Autodesk Fusion 360 part; units mm, degrees
(part 2 of 3)
sketch "Sketch5" plane through (0, 0, 0) normal (0, 0, -1) x (1, 0, 0)
  arc A0 (13.748372, 9.324199) -> (13.417296, 7.858359) centre (14.366478, 8.414284) ccw
  line L0 (13.748372, 9.324199) -> (13.998575, 9.494162)
  spline S0 degree 5 poles (13.998575, 9.494162) (14.006089, 9.499267) (14.020968, 9.509672) (14.042834, 9.52587) (14.071131, 9.54859) (14.10533, 9.578527) (14.138686, 9.609581) (14.171524, 9.641334) (14.204082, 9.673474) (14.236451, 9.70588) (14.26862, 9.738556) (14.300516, 9.771583) (14.33205, 9.805066) (14.363159, 9.839079) (14.39384, 9.873623) (14.424122, 9.908656) (14.454056, 9.944111) (14.483697, 9.97992) (14.513083, 10.016032) (14.542226, 10.052428) (14.571122, 10.089111) (14.599759, 10.126094) (14.628121, 10.163392) (14.656202, 10.201013) (14.684003, 10.238952) (14.711532, 10.277197) (14.7388, 10.315731) (14.76582, 10.35454) (14.792599, 10.39361) (14.819141, 10.432935) (14.845446, 10.472514) (14.871513, 10.512344) (14.897342, 10.552427) (14.922931, 10.59276) (14.948283, 10.63334) (14.9734, 10.674162) (14.998286, 10.71522) (15.022944, 10.756508) (15.047376, 10.798023) (15.071584, 10.83976) (15.095569, 10.881717) (15.119331, 10.923891) (15.142871, 10.966281) (15.16619, 11.008883) (15.189289, 11.051696) (15.212169, 11.094715) (15.234832, 11.137939) (15.257278, 11.181365) (15.279509, 11.224989) (15.301525, 11.268809) (15.323328, 11.312823) (15.344917, 11.357029) (15.366295, 11.401425) (15.38746, 11.446008) (15.408415, 11.490777) (15.429159, 11.53573) (15.449693, 11.580863) (15.470018, 11.626176) (15.490134, 11.671666) (15.510043, 11.717332) (15.529744, 11.763171) (15.549238, 11.809183) (15.568525, 11.855365) (15.587606, 11.901715) (15.606482, 11.948232) (15.625151, 11.994914) (15.643616, 12.041758) (15.661877, 12.088763) (15.679933, 12.135927) (15.697785, 12.18325) (15.715433, 12.230731) (15.72939, 12.268841) (15.739766, 12.297494) (15.746643, 12.316628) (15.750071, 12.326202) knots 0 0 0 0 0 0 0.01428571 0.02857143 0.04285714 0.05714286 0.07142857 0.08571429 0.1 0.11428571 0.12857143 0.14285714 0.15714286 0.17142857 0.18571429 0.2 0.21428571 0.22857143 0.24285714 0.25714286 0.27142857 0.28571429 0.3 0.31428571 0.32857143 0.34285714 0.35714286 0.37142857 0.38571429 0.4 0.41428571 0.42857143 0.44285714 0.45714286 0.47142857 0.48571429 0.5 0.51428571 0.52857143 0.54285714 0.55714286 0.57142857 0.58571429 0.6 0.61428571 0.62857143 0.64285714 0.65714286 0.67142857 0.68571429 0.7 0.71428571 0.72857143 0.74285714 0.75714286 0.77142857 0.78571429 0.8 0.81428571 0.82857143 0.84285714 0.85714286 0.87142857 0.88571429 0.9 0.91428571 0.92857143 0.94285714 0.95714286 0.97142857 0.98571429 1 1 1 1 1 1
  arc A1 (15.750071, 12.326202) -> (14.873911, 13.37037) centre (0, 0) ccw
  spline S1 degree 5 poles (11.780751, 12.137261) (11.787083, 12.143775) (11.799915, 12.15662) (11.819664, 12.175342) (11.846951, 12.199263) (11.882373, 12.227744) (11.918747, 12.255201) (11.95572, 12.282026) (11.993026, 12.308509) (12.03056, 12.334759) (12.068325, 12.360765) (12.106389, 12.386441) (12.14484, 12.411682) (12.183738, 12.436412) (12.223084, 12.460628) (12.262843, 12.484367) (12.302959, 12.50769) (12.34337, 12.530663) (12.384036, 12.553331) (12.42494, 12.575711) (12.466084, 12.597798) (12.507477, 12.619578) (12.549133, 12.641033) (12.591059, 12.662154) (12.633249, 12.682945) (12.675694, 12.703414) (12.718378, 12.723577) (12.761289, 12.743447) (12.804415, 12.763035) (12.847752, 12.782345) (12.891297, 12.801377) (12.935049, 12.820132) (12.979008, 12.838608) (13.023172, 12.856805) (13.067538, 12.874725) (13.112101, 12.892372) (13.156857, 12.90975) (13.2018, 12.926864) (13.246926, 12.943716) (13.292233, 12.960308) (13.337717, 12.976643) (13.383377, 12.992721) (13.42921, 13.008542) (13.475215, 13.024109) (13.521388, 13.039423) (13.567727, 13.054485) (13.61423, 13.069298) (13.660893, 13.083862) (13.707715, 13.09818) (13.754692, 13.112252) (13.801824, 13.126081) (13.849107, 13.139666) (13.896541, 13.15301) (13.944122, 13.166112) (13.99185, 13.178974) (14.039721, 13.191597) (14.087735, 13.203982) (14.135889, 13.216129) (14.184181, 13.228041) (14.23261, 13.239717) (14.281174, 13.251159) (14.329872, 13.262367) (14.378701, 13.273342) (14.427661, 13.284084) (14.476749, 13.294595) (14.525963, 13.304875) (14.575302, 13.314925) (14.624764, 13.324746) (14.674347, 13.334337) (14.724051, 13.343701) (14.773875, 13.352836) (14.81383, 13.359963) (14.843849, 13.365206) (14.863886, 13.368656) (14.873911, 13.37037) knots 0 0 0 0 0 0 0.01428571 0.02857143 0.04285714 0.05714286 0.07142857 0.08571429 0.1 0.11428571 0.12857143 0.14285714 0.15714286 0.17142857 0.18571429 0.2 0.21428571 0.22857143 0.24285714 0.25714286 0.27142857 0.28571429 0.3 0.31428571 0.32857143 0.34285714 0.35714286 0.37142857 0.38571429 0.4 0.41428571 0.42857143 0.44285714 0.45714286 0.47142857 0.48571429 0.5 0.51428571 0.52857143 0.54285714 0.55714286 0.57142857 0.58571429 0.6 0.61428571 0.62857143 0.64285714 0.65714286 0.67142857 0.68571429 0.7 0.71428571 0.72857143 0.74285714 0.75714286 0.77142857 0.78571429 0.8 0.81428571 0.82857143 0.84285714 0.85714286 0.87142857 0.88571429 0.9 0.91428571 0.92857143 0.94285714 0.95714286 0.97142857 0.98571429 1 1 1 1 1 1
  line L1 (11.780751, 12.137261) -> (11.569923, 11.920373)
  arc A2 (10.068861, 11.848867) -> (11.569923, 11.920373) centre (10.781165, 12.687094) ccw
  arc A3 (10.068861, 11.848867) -> (9.920417, 11.973427) centre (0, 0) ccw
  arc A4 (9.73018, 13.464101) -> (9.920417, 11.973427) centre (10.622219, 12.820465) ccw
  line L2 (9.73018, 13.464101) -> (9.907163, 13.709388)
  spline S2 degree 5 poles (9.907163, 13.709388) (9.912478, 13.716755) (9.9229, 13.731622) (9.937908, 13.754322) (9.956728, 13.785349) (9.978625, 13.825178) (9.999348, 13.865768) (10.019346, 13.906837) (10.038948, 13.948175) (10.058282, 13.989697) (10.077334, 14.031405) (10.096011, 14.073349) (10.114191, 14.115598) (10.131791, 14.1582) (10.148807, 14.201154) (10.165281, 14.244431) (10.181284, 14.287987) (10.19689, 14.331774) (10.212152, 14.375758) (10.227089, 14.419927) (10.241697, 14.46428) (10.255957, 14.508827) (10.269853, 14.553576) (10.283373, 14.598532) (10.296521, 14.643692) (10.30931, 14.689046) (10.321754, 14.734583) (10.333871, 14.780293) (10.345672, 14.826165) (10.357163, 14.872197) (10.368345, 14.918385) (10.379218, 14.964729) (10.389779, 15.011229) (10.400031, 15.057882) (10.409975, 15.104685) (10.419615, 15.151636) (10.428958, 15.198729) (10.438007, 15.245961) (10.446767, 15.293328) (10.45524, 15.340828) (10.463428, 15.388457) (10.471333, 15.436215) (10.478955, 15.4841) (10.486297, 15.532109) (10.493361, 15.58024) (10.500147, 15.62849) (10.506659, 15.676859) (10.5129, 15.725342) (10.518869, 15.773939) (10.524571, 15.822646) (10.530005, 15.871463) (10.535173, 15.920387) (10.540077, 15.969417) (10.544718, 16.018551) (10.549096, 16.067787) (10.553215, 16.117123) (10.557074, 16.166558) (10.560675, 16.21609) (10.56402, 16.265717) (10.567109, 16.315437) (10.569944, 16.36525) (10.572525, 16.415154) (10.574854, 16.465148) (10.576932, 16.515229) (10.578759, 16.565397) (10.580338, 16.615648) (10.581667, 16.665983) (10.582749, 16.716399) (10.583585, 16.766894) (10.584175, 16.817469) (10.58452, 16.868122) (10.584601, 16.908708) (10.584551, 16.939182) (10.584469, 16.959513) (10.584416, 16.969683) knots 0 0 0 0 0 0 0.01428571 0.02857143 0.04285714 0.05714286 0.07142857 0.08571429 0.1 0.11428571 0.12857143 0.14285714 0.15714286 0.17142857 0.18571429 0.2 0.21428571 0.22857143 0.24285714 0.25714286 0.27142857 0.28571429 0.3 0.31428571 0.32857143 0.34285714 0.35714286 0.37142857 0.38571429 0.4 0.41428571 0.42857143 0.44285714 0.45714286 0.47142857 0.48571429 0.5 0.51428571 0.52857143 0.54285714 0.55714286 0.57142857 0.58571429 0.6 0.61428571 0.62857143 0.64285714 0.65714286 0.67142857 0.68571429 0.7 0.71428571 0.72857143 0.74285714 0.75714286 0.77142857 0.78571429 0.8 0.81428571 0.82857143 0.84285714 0.85714286 0.87142857 0.88571429 0.9 0.91428571 0.92857143 0.94285714 0.95714286 0.97142857 0.98571429 1 1 1 1 1 1
  arc A5 (10.584416, 16.969683) -> (9.403968, 17.651215) centre (0, 0) ccw
  spline S3 degree 5 poles (6.919097, 15.434549) (6.922819, 15.442835) (6.930484, 15.459295) (6.942639, 15.483642) (6.960099, 15.515454) (6.983643, 15.554332) (7.008433, 15.592574) (7.034001, 15.630426) (7.06, 15.668072) (7.086292, 15.705576) (7.112886, 15.74293) (7.139872, 15.780076) (7.167371, 15.816946) (7.195465, 15.853489) (7.224156, 15.889701) (7.253398, 15.925607) (7.283117, 15.961244) (7.313235, 15.996652) (7.343695, 16.031862) (7.374478, 16.066883) (7.405586, 16.10171) (7.437034, 16.136333) (7.46884, 16.170742) (7.501013, 16.204929) (7.533549, 16.238895) (7.566432, 16.272647) (7.599646, 16.306193) (7.633173, 16.339541) (7.667, 16.372698) (7.701119, 16.405665) (7.735528, 16.438443) (7.770227, 16.471031) (7.805216, 16.503427) (7.840493, 16.535632) (7.876054, 16.567645) (7.911894, 16.59947) (7.948007, 16.631107) (7.984386, 16.66256) (8.021027, 16.69383) (8.057926, 16.724917) (8.095081, 16.755823) (8.132488, 16.786548) (8.170146, 16.817092) (8.208052, 16.847454) (8.246203, 16.877637) (8.284596, 16.907639) (8.323228, 16.937463) (8.362096, 16.967109) (8.401197, 16.996577) (8.440528, 17.025869) (8.480088, 17.054983) (8.519873, 17.083921) (8.559882, 17.112683) (8.600113, 17.141269) (8.640563, 17.169679) (8.681231, 17.197914) (8.722113, 17.225973) (8.763208, 17.253858) (8.804514, 17.281568) (8.846029, 17.309104) (8.887751, 17.336465) (8.929678, 17.363653) (8.971809, 17.390667) (9.014142, 17.417506) (9.056674, 17.444173) (9.099405, 17.470665) (9.142331, 17.496984) (9.185451, 17.523129) (9.228764, 17.549101) (9.272268, 17.574899) (9.315962, 17.600525) (9.35107, 17.620887) (9.377486, 17.636081) (9.395135, 17.646176) (9.403968, 17.651215) knots 0 0 0 0 0 0 0.01428571 0.02857143 0.04285714 0.05714286 0.07142857 0.08571429 0.1 0.11428571 0.12857143 0.14285714 0.15714286 0.17142857 0.18571429 0.2 0.21428571 0.22857143 0.24285714 0.25714286 0.27142857 0.28571429 0.3 0.31428571 0.32857143 0.34285714 0.35714286 0.37142857 0.38571429 0.4 0.41428571 0.42857143 0.44285714 0.45714286 0.47142857 0.48571429 0.5 0.51428571 0.52857143 0.54285714 0.55714286 0.57142857 0.58571429 0.6 0.61428571 0.62857143 0.64285714 0.65714286 0.67142857 0.68571429 0.7 0.71428571 0.72857143 0.74285714 0.75714286 0.77142857 0.78571429 0.8 0.81428571 0.82857143 0.84285714 0.85714286 0.87142857 0.88571429 0.9 0.91428571 0.92857143 0.94285714 0.95714286 0.97142857 0.98571429 1 1 1 1 1 1
  line L3 (6.919097, 15.434549) -> (6.795164, 15.158633)
  arc A6 (5.409084, 14.578046) -> (6.795164, 15.158633) centre (5.791739, 15.609344) ccw
  arc A7 (5.409084, 14.578046) -> (5.226989, 14.644323) centre (0, 0) ccw
  arc A8 (4.538384, 15.980034) -> (5.226989, 14.644323) centre (5.596763, 15.680309) ccw
  line L4 (4.538384, 15.980034) -> (4.620801, 16.27106)
  spline S4 degree 5 poles (4.620801, 16.27106) (4.623276, 16.279801) (4.627985, 16.297336) (4.634323, 16.3238) (4.641396, 16.359393) (4.648351, 16.404309) (4.653942, 16.449538) (4.658687, 16.49497) (4.662969, 16.54052) (4.666935, 16.58615) (4.670574, 16.631859) (4.673778, 16.677661) (4.676412, 16.72358) (4.67838, 16.769633) (4.679678, 16.815816) (4.680357, 16.862117) (4.680498, 16.90852) (4.680187, 16.955004) (4.679486, 17.001556) (4.678415, 17.048169) (4.676971, 17.094844) (4.675136, 17.141582) (4.672889, 17.188385) (4.670218, 17.235254) (4.667128, 17.282187) (4.663633, 17.32918) (4.659752, 17.376227) (4.655505, 17.423324) (4.650905, 17.470467) (4.645959, 17.517652) (4.640669, 17.56488) (4.635035, 17.612147) (4.629056, 17.659455) (4.622733, 17.7068) (4.61607, 17.754182) (4.609071, 17.801599) (4.601743, 17.849047) (4.594093, 17.896526) (4.586124, 17.944032) (4.57784, 17.991565) (4.569244, 18.039123) (4.560338, 18.086705) (4.551123, 18.134308) (4.541602, 18.181933) (4.531778, 18.229577) (4.521652, 18.277239) (4.511229, 18.324918) (4.50051, 18.372611) (4.489499, 18.420319) (4.478198, 18.468039) (4.466608, 18.51577) (4.454731, 18.563512) (4.44257, 18.611262) (4.430126, 18.65902) (4.417401, 18.706784) (4.404397, 18.754554) (4.391116, 18.802327) (4.377559, 18.850103) (4.363729, 18.897881) (4.349626, 18.94566) (4.335253, 18.993439) (4.320611, 19.041216) (4.305701, 19.088991) (4.290524, 19.136763) (4.275083, 19.18453) (4.259379, 19.232291) (4.243413, 19.280044) (4.227187, 19.32779) (4.210701, 19.375526) (4.193958, 19.423253) (4.176958, 19.470969) (4.163153, 19.509134) (4.152683, 19.537754) (4.145653, 19.556831) (4.142124, 19.566369) knots 0 0 0 0 0 0 0.01428571 0.02857143 0.04285714 0.05714286 0.07142857 0.08571429 0.1 0.11428571 0.12857143 0.14285714 0.15714286 0.17142857 0.18571429 0.2 0.21428571 0.22857143 0.24285714 0.25714286 0.27142857 0.28571429 0.3 0.31428571 0.32857143 0.34285714 0.35714286 0.37142857 0.38571429 0.4 0.41428571 0.42857143 0.44285714 0.45714286 0.47142857 0.48571429 0.5 0.51428571 0.52857143 0.54285714 0.55714286 0.57142857 0.58571429 0.6 0.61428571 0.62857143 0.64285714 0.65714286 0.67142857 0.68571429 0.7 0.71428571 0.72857143 0.74285714 0.75714286 0.77142857 0.78571429 0.8 0.81428571 0.82857143 0.84285714 0.85714286 0.87142857 0.88571429 0.9 0.91428571 0.92857143 0.94285714 0.95714286 0.97142857 0.98571429 1 1 1 1 1 1
  arc A9 (4.142124, 19.566369) -> (2.799769, 19.803063) centre (0, 0) ccw
  spline S5 degree 5 poles (1.222898, 16.870202) (1.223562, 16.879262) (1.225134, 16.89735) (1.228229, 16.924386) (1.233756, 16.960251) (1.242583, 17.004837) (1.252798, 17.049252) (1.263878, 17.093567) (1.275433, 17.137833) (1.287313, 17.182069) (1.299527, 17.226265) (1.312181, 17.270401) (1.325412, 17.314452) (1.339313, 17.3584) (1.353888, 17.402242) (1.369087, 17.445984) (1.384825, 17.489636) (1.401016, 17.53321) (1.417596, 17.576715) (1.434545, 17.620151) (1.451866, 17.663517) (1.469575, 17.706809) (1.487695, 17.75002) (1.506235, 17.79315) (1.525191, 17.836195) (1.544547, 17.879159) (1.564285, 17.922041) (1.584385, 17.964845) (1.604831, 18.007572) (1.625617, 18.05022) (1.64674, 18.09279) (1.668201, 18.13528) (1.689999, 18.17769) (1.712134, 18.220017) (1.734601, 18.262263) (1.757395, 18.304426) (1.780509, 18.346507) (1.803937, 18.388505) (1.827674, 18.430421) (1.851715, 18.472255) (1.876059, 18.514004) (1.900702, 18.55567) (1.925642, 18.597251) (1.950877, 18.638748) (1.976404, 18.680158) (2.002221, 18.721483) (2.028322, 18.762721) (2.054707, 18.803873) (2.081371, 18.844937) (2.108312, 18.885914) (2.135528, 18.926803) (2.163017, 18.967603) (2.190776, 19.008314) (2.218804, 19.048936) (2.247098, 19.089467) (2.275656, 19.129908) (2.304475, 19.170258) (2.333555, 19.210517) (2.362892, 19.250683) (2.392486, 19.290757) (2.422333, 19.330738) (2.452433, 19.370626) (2.482784, 19.41042) (2.513385, 19.45012) (2.544232, 19.489725) (2.575324, 19.529235) (2.60666, 19.568648) (2.638237, 19.607964) (2.670055, 19.647184) (2.702112, 19.686306) (2.734407, 19.72533) (2.760433, 19.756472) (2.780059, 19.779784) (2.793191, 19.795307) (2.799769, 19.803063) knots 0 0 0 0 0 0 0.01428571 0.02857143 0.04285714 0.05714286 0.07142857 0.08571429 0.1 0.11428571 0.12857143 0.14285714 0.15714286 0.17142857 0.18571429 0.2 0.21428571 0.22857143 0.24285714 0.25714286 0.27142857 0.28571429 0.3 0.31428571 0.32857143 0.34285714 0.35714286 0.37142857 0.38571429 0.4 0.41428571 0.42857143 0.44285714 0.45714286 0.47142857 0.48571429 0.5 0.51428571 0.52857143 0.54285714 0.55714286 0.57142857 0.58571429 0.6 0.61428571 0.62857143 0.64285714 0.65714286 0.67142857 0.68571429 0.7 0.71428571 0.72857143 0.74285714 0.75714286 0.77142857 0.78571429 0.8 0.81428571 0.82857143 0.84285714 0.85714286 0.87142857 0.88571429 0.9 0.91428571 0.92857143 0.94285714 0.95714286 0.97142857 0.98571429 1 1 1 1 1 1
  line L5 (1.222898, 16.870202) -> (1.200807, 16.568538)
  arc A10 (0.09689, 15.548898) -> (1.200807, 16.568538) centre (0.103745, 16.648877) ccw
  arc A11 (0.09689, 15.548898) -> (-0.09689, 15.548898) centre (0, 0) ccw
  arc A12 (-1.200807, 16.568538) -> (-0.09689, 15.548898) centre (-0.103745, 16.648877) ccw
  line L6 (-1.200807, 16.568538) -> (-1.222898, 16.870202)
  spline S6 degree 5 poles (-1.222898, 16.870202) (-1.223562, 16.879262) (-1.225134, 16.89735) (-1.228229, 16.924386) (-1.233756, 16.960251) (-1.242583, 17.004837) (-1.252798, 17.049252) (-1.263878, 17.093567) (-1.275433, 17.137833) (-1.287313, 17.182069) (-1.299527, 17.226265) (-1.312181, 17.270401) (-1.325412, 17.314452) (-1.339313, 17.3584) (-1.353888, 17.402242) (-1.369087, 17.445984) (-1.384825, 17.489636) (-1.401016, 17.53321) (-1.417596, 17.576715) (-1.434545, 17.620151) (-1.451866, 17.663517) (-1.469575, 17.706809) (-1.487695, 17.75002) (-1.506235, 17.79315) (-1.525191, 17.836195) (-1.544547, 17.879159) (-1.564285, 17.922041) (-1.584385, 17.964845) (-1.604831, 18.007572) (-1.625617, 18.05022) (-1.64674, 18.09279) (-1.668201, 18.13528) (-1.689999, 18.17769) (-1.712134, 18.220017) (-1.734601, 18.262263) (-1.757395, 18.304426) (-1.780509, 18.346507) (-1.803937, 18.388505) (-1.827674, 18.430421) (-1.851715, 18.472255) (-1.876059, 18.514004) (-1.900702, 18.55567) (-1.925642, 18.597251) (-1.950877, 18.638748) (-1.976404, 18.680158) (-2.002221, 18.721483) (-2.028322, 18.762721) (-2.054707, 18.803873) (-2.081371, 18.844937) (-2.108312, 18.885914) (-2.135528, 18.926803) (-2.163017, 18.967603) (-2.190776, 19.008314) (-2.218804, 19.048936) (-2.247098, 19.089467) (-2.275656, 19.129908) (-2.304475, 19.170258) (-2.333555, 19.210517) (-2.362892, 19.250683) (-2.392486, 19.290757) (-2.422333, 19.330738) (-2.452433, 19.370626) (-2.482784, 19.41042) (-2.513385, 19.45012) (-2.544232, 19.489725) (-2.575324, 19.529235) (-2.60666, 19.568648) (-2.638237, 19.607964) (-2.670055, 19.647184) (-2.702112, 19.686306) (-2.734407, 19.72533) (-2.760433, 19.756472) (-2.780059, 19.779784) (-2.793191, 19.795307) (-2.799769, 19.803063) knots 0 0 0 0 0 0 0.01428571 0.02857143 0.04285714 0.05714286 0.07142857 0.08571429 0.1 0.11428571 0.12857143 0.14285714 0.15714286 0.17142857 0.18571429 0.2 0.21428571 0.22857143 0.24285714 0.25714286 0.27142857 0.28571429 0.3 0.31428571 0.32857143 0.34285714 0.35714286 0.37142857 0.38571429 0.4 0.41428571 0.42857143 0.44285714 0.45714286 0.47142857 0.48571429 0.5 0.51428571 0.52857143 0.54285714 0.55714286 0.57142857 0.58571429 0.6 0.61428571 0.62857143 0.64285714 0.65714286 0.67142857 0.68571429 0.7 0.71428571 0.72857143 0.74285714 0.75714286 0.77142857 0.78571429 0.8 0.81428571 0.82857143 0.84285714 0.85714286 0.87142857 0.88571429 0.9 0.91428571 0.92857143 0.94285714 0.95714286 0.97142857 0.98571429 1 1 1 1 1 1
  arc A13 (-2.799769, 19.803063) -> (-4.142124, 19.566369) centre (0, 0) ccw
  spline S7 degree 5 poles (-4.620801, 16.27106) (-4.623276, 16.279801) (-4.627985, 16.297336) (-4.634323, 16.3238) (-4.641396, 16.359393) (-4.648351, 16.404309) (-4.653942, 16.449538) (-4.658687, 16.49497) (-4.662969, 16.54052) (-4.666935, 16.58615) (-4.670574, 16.631859) (-4.673778, 16.677661) (-4.676412, 16.72358) (-4.67838, 16.769633) (-4.679678, 16.815816) (-4.680357, 16.862117) (-4.680498, 16.90852) (-4.680187, 16.955004) (-4.679486, 17.001556) (-4.678415, 17.048169) (-4.676971, 17.094844) (-4.675136, 17.141582) (-4.672889, 17.188385) (-4.670218, 17.235254) (-4.667128, 17.282187) (-4.663633, 17.32918) (-4.659752, 17.376227) (-4.655505, 17.423324) (-4.650905, 17.470467) (-4.645959, 17.517652) (-4.640669, 17.56488) (-4.635035, 17.612147) (-4.629056, 17.659455) (-4.622733, 17.7068) (-4.61607, 17.754182) (-4.609071, 17.801599) (-4.601743, 17.849047) (-4.594093, 17.896526) (-4.586124, 17.944032) (-4.57784, 17.991565) (-4.569244, 18.039123) (-4.560338, 18.086705) (-4.551123, 18.134308) (-4.541602, 18.181933) (-4.531778, 18.229577) (-4.521652, 18.277239) (-4.511229, 18.324918) (-4.50051, 18.372611) (-4.489499, 18.420319) (-4.478198, 18.468039) (-4.466608, 18.51577) (-4.454731, 18.563512) (-4.44257, 18.611262) (-4.430126, 18.65902) (-4.417401, 18.706784) (-4.404397, 18.754554) (-4.391116, 18.802327) (-4.377559, 18.850103) (-4.363729, 18.897881) (-4.349626, 18.94566) (-4.335253, 18.993439) (-4.320611, 19.041216) (-4.305701, 19.088991) (-4.290524, 19.136763) (-4.275083, 19.18453) (-4.259379, 19.232291) (-4.243413, 19.280044) (-4.227187, 19.32779) (-4.210701, 19.375526) (-4.193958, 19.423253) (-4.176958, 19.470969) (-4.163153, 19.509134) (-4.152683, 19.537754) (-4.145653, 19.556831) (-4.142124, 19.566369) knots 0 0 0 0 0 0 0.01428571 0.02857143 0.04285714 0.05714286 0.07142857 0.08571429 0.1 0.11428571 0.12857143 0.14285714 0.15714286 0.17142857 0.18571429 0.2 0.21428571 0.22857143 0.24285714 0.25714286 0.27142857 0.28571429 0.3 0.31428571 0.32857143 0.34285714 0.35714286 0.37142857 0.38571429 0.4 0.41428571 0.42857143 0.44285714 0.45714286 0.47142857 0.48571429 0.5 0.51428571 0.52857143 0.54285714 0.55714286 0.57142857 0.58571429 0.6 0.61428571 0.62857143 0.64285714 0.65714286 0.67142857 0.68571429 0.7 0.71428571 0.72857143 0.74285714 0.75714286 0.77142857 0.78571429 0.8 0.81428571 0.82857143 0.84285714 0.85714286 0.87142857 0.88571429 0.9 0.91428571 0.92857143 0.94285714 0.95714286 0.97142857 0.98571429 1 1 1 1 1 1
  line L7 (-4.620801, 16.27106) -> (-4.538384, 15.980034)
  arc A14 (-5.226989, 14.644323) -> (-4.538384, 15.980034) centre (-5.596763, 15.680309) ccw
  arc A15 (-5.226989, 14.644323) -> (-5.409084, 14.578046) centre (0, 0) ccw
  arc A16 (-6.795164, 15.158633) -> (-5.409084, 14.578046) centre (-5.791739, 15.609344) ccw
  line L8 (-6.795164, 15.158633) -> (-6.919097, 15.434549)
  spline S8 degree 5 poles (-6.919097, 15.434549) (-6.922819, 15.442835) (-6.930484, 15.459295) (-6.942639, 15.483642) (-6.960099, 15.515454) (-6.983643, 15.554332) (-7.008433, 15.592574) (-7.034001, 15.630426) (-7.06, 15.668072) (-7.086292, 15.705576) (-7.112886, 15.74293) (-7.139872, 15.780076) (-7.167371, 15.816946) (-7.195465, 15.853489) (-7.224156, 15.889701) (-7.253398, 15.925607) (-7.283117, 15.961244) (-7.313235, 15.996652) (-7.343695, 16.031862) (-7.374478, 16.066883) (-7.405586, 16.10171) (-7.437034, 16.136333) (-7.46884, 16.170742) (-7.501013, 16.204929) (-7.533549, 16.238895) (-7.566432, 16.272647) (-7.599646, 16.306193) (-7.633173, 16.339541) (-7.667, 16.372698) (-7.701119, 16.405665) (-7.735528, 16.438443) (-7.770227, 16.471031) (-7.805216, 16.503427) (-7.840493, 16.535632) (-7.876054, 16.567645) (-7.911894, 16.59947) (-7.948007, 16.631107) (-7.984386, 16.66256) (-8.021027, 16.69383) (-8.057926, 16.724917) (-8.095081, 16.755823) (-8.132488, 16.786548) (-8.170146, 16.817092) (-8.208052, 16.847454) (-8.246203, 16.877637) (-8.284596, 16.907639) (-8.323228, 16.937463) (-8.362096, 16.967109) (-8.401197, 16.996577) (-8.440528, 17.025869) (-8.480088, 17.054983) (-8.519873, 17.083921) (-8.559882, 17.112683) (-8.600113, 17.141269) (-8.640563, 17.169679) (-8.681231, 17.197914) (-8.722113, 17.225973) (-8.763208, 17.253858) (-8.804514, 17.281568) (-8.846029, 17.309104) (-8.887751, 17.336465) (-8.929678, 17.363653) (-8.971809, 17.390667) (-9.014142, 17.417506) (-9.056674, 17.444173) (-9.099405, 17.470665) (-9.142331, 17.496984) (-9.185451, 17.523129) (-9.228764, 17.549101) (-9.272268, 17.574899) (-9.315962, 17.600525) (-9.35107, 17.620887) (-9.377486, 17.636081) (-9.395135, 17.646176) (-9.403968, 17.651215) knots 0 0 0 0 0 0 0.01428571 0.02857143 0.04285714 0.05714286 0.07142857 0.08571429 0.1 0.11428571 0.12857143 0.14285714 0.15714286 0.17142857 0.18571429 0.2 0.21428571 0.22857143 0.24285714 0.25714286 0.27142857 0.28571429 0.3 0.31428571 0.32857143 0.34285714 0.35714286 0.37142857 0.38571429 0.4 0.41428571 0.42857143 0.44285714 0.45714286 0.47142857 0.48571429 0.5 0.51428571 0.52857143 0.54285714 0.55714286 0.57142857 0.58571429 0.6 0.61428571 0.62857143 0.64285714 0.65714286 0.67142857 0.68571429 0.7 0.71428571 0.72857143 0.74285714 0.75714286 0.77142857 0.78571429 0.8 0.81428571 0.82857143 0.84285714 0.85714286 0.87142857 0.88571429 0.9 0.91428571 0.92857143 0.94285714 0.95714286 0.97142857 0.98571429 1 1 1 1 1 1
  arc A17 (-9.403968, 17.651215) -> (-10.584416, 16.969683) centre (0, 0) ccw
  spline S9 degree 5 poles (-9.907163, 13.709388) (-9.912478, 13.716755) (-9.9229, 13.731622) (-9.937908, 13.754322) (-9.956728, 13.785349) (-9.978625, 13.825178) (-9.999348, 13.865768) (-10.019346, 13.906837) (-10.038948, 13.948175) (-10.058282, 13.989697) (-10.077334, 14.031405) (-10.096011, 14.073349) (-10.114191, 14.115598) (-10.131791, 14.1582) (-10.148807, 14.201154) (-10.165281, 14.244431) (-10.181284, 14.287987) (-10.19689, 14.331774) (-10.212152, 14.375758) (-10.227089, 14.419927) (-10.241697, 14.46428) (-10.255957, 14.508827) (-10.269853, 14.553576) (-10.283373, 14.598532) (-10.296521, 14.643692) (-10.30931, 14.689046) (-10.321754, 14.734583) (-10.333871, 14.780293) (-10.345672, 14.826165) (-10.357163, 14.872197) (-10.368345, 14.918385) (-10.379218, 14.964729) (-10.389779, 15.011229) (-10.400031, 15.057882) (-10.409975, 15.104685) (-10.419615, 15.151636) (-10.428958, 15.198729) (-10.438007, 15.245961) (-10.446767, 15.293328) (-10.45524, 15.340828) (-10.463428, 15.388457) (-10.471333, 15.436215) (-10.478955, 15.4841) (-10.486297, 15.532109) (-10.493361, 15.58024) (-10.500147, 15.62849) (-10.506659, 15.676859) (-10.5129, 15.725342) (-10.518869, 15.773939) (-10.524571, 15.822646) (-10.530005, 15.871463) (-10.535173, 15.920387) (-10.540077, 15.969417) (-10.544718, 16.018551) (-10.549096, 16.067787) (-10.553215, 16.117123) (-10.557074, 16.166558) (-10.560675, 16.21609) (-10.56402, 16.265717) (-10.567109, 16.315437) (-10.569944, 16.36525) (-10.572525, 16.415154) (-10.574854, 16.465148) (-10.576932, 16.515229) (-10.578759, 16.565397) (-10.580338, 16.615648) (-10.581667, 16.665983) (-10.582749, 16.716399) (-10.583585, 16.766894) (-10.584175, 16.817469) (-10.58452, 16.868122) (-10.584601, 16.908708) (-10.584551, 16.939182) (-10.584469, 16.959513) (-10.584416, 16.969683) knots 0 0 0 0 0 0 0.01428571 0.02857143 0.04285714 0.05714286 0.07142857 0.08571429 0.1 0.11428571 0.12857143 0.14285714 0.15714286 0.17142857 0.18571429 0.2 0.21428571 0.22857143 0.24285714 0.25714286 0.27142857 0.28571429 0.3 0.31428571 0.32857143 0.34285714 0.35714286 0.37142857 0.38571429 0.4 0.41428571 0.42857143 0.44285714 0.45714286 0.47142857 0.48571429 0.5 0.51428571 0.52857143 0.54285714 0.55714286 0.57142857 0.58571429 0.6 0.61428571 0.62857143 0.64285714 0.65714286 0.67142857 0.68571429 0.7 0.71428571 0.72857143 0.74285714 0.75714286 0.77142857 0.78571429 0.8 0.81428571 0.82857143 0.84285714 0.85714286 0.87142857 0.88571429 0.9 0.91428571 0.92857143 0.94285714 0.95714286 0.97142857 0.98571429 1 1 1 1 1 1
  line L9 (-9.907163, 13.709388) -> (-9.73018, 13.464101)
  arc A18 (-9.920417, 11.973427) -> (-9.73018, 13.464101) centre (-10.622219, 12.820465) ccw
  arc A19 (-9.920417, 11.973427) -> (-10.068861, 11.848867) centre (0, 0) ccw
  arc A20 (-11.569923, 11.920373) -> (-10.068861, 11.848867) centre (-10.781165, 12.687094) ccw
  line L10 (-11.569923, 11.920373) -> (-11.780751, 12.137261)
  spline S10 degree 5 poles (-11.780751, 12.137261) (-11.787083, 12.143775) (-11.799915, 12.15662) (-11.819664, 12.175342) (-11.846951, 12.199263) (-11.882373, 12.227744) (-11.918747, 12.255201) (-11.95572, 12.282026) (-11.993026, 12.308509) (-12.03056, 12.334759) (-12.068325, 12.360765) (-12.106389, 12.386441) (-12.14484, 12.411682) (-12.183738, 12.436412) (-12.223084, 12.460628) (-12.262843, 12.484367) (-12.302959, 12.50769) (-12.34337, 12.530663) (-12.384036, 12.553331) (-12.42494, 12.575711) (-12.466084, 12.597798) (-12.507477, 12.619578) (-12.549133, 12.641033) (-12.591059, 12.662154) (-12.633249, 12.682945) (-12.675694, 12.703414) (-12.718378, 12.723577) (-12.761289, 12.743447) (-12.804415, 12.763035) (-12.847752, 12.782345) (-12.891297, 12.801377) (-12.935049, 12.820132) (-12.979008, 12.838608) (-13.023172, 12.856805) (-13.067538, 12.874725) (-13.112101, 12.892372) (-13.156857, 12.90975) (-13.2018, 12.926864) (-13.246926, 12.943716) (-13.292233, 12.960308) (-13.337717, 12.976643) (-13.383377, 12.992721) (-13.42921, 13.008542) (-13.475215, 13.024109) (-13.521388, 13.039423) (-13.567727, 13.054485) (-13.61423, 13.069298) (-13.660893, 13.083862) (-13.707715, 13.09818) (-13.754692, 13.112252) (-13.801824, 13.126081) (-13.849107, 13.139666) (-13.896541, 13.15301) (-13.944122, 13.166112) (-13.99185, 13.178974) (-14.039721, 13.191597) (-14.087735, 13.203982) (-14.135889, 13.216129) (-14.184181, 13.228041) (-14.23261, 13.239717) (-14.281174, 13.251159) (-14.329872, 13.262367) (-14.378701, 13.273342) (-14.427661, 13.284084) (-14.476749, 13.294595) (-14.525963, 13.304875) (-14.575302, 13.314925) (-14.624764, 13.324746) (-14.674347, 13.334337) (-14.724051, 13.343701) (-14.773875, 13.352836) (-14.81383, 13.359963) (-14.843849, 13.365206) (-14.863886, 13.368656) (-14.873911, 13.37037) knots 0 0 0 0 0 0 0.01428571 0.02857143 0.04285714 0.05714286 0.07142857 0.08571429 0.1 0.11428571 0.12857143 0.14285714 0.15714286 0.17142857 0.18571429 0.2 0.21428571 0.22857143 0.24285714 0.25714286 0.27142857 0.28571429 0.3 0.31428571 0.32857143 0.34285714 0.35714286 0.37142857 0.38571429 0.4 0.41428571 0.42857143 0.44285714 0.45714286 0.47142857 0.48571429 0.5 0.51428571 0.52857143 0.54285714 0.55714286 0.57142857 0.58571429 0.6 0.61428571 0.62857143 0.64285714 0.65714286 0.67142857 0.68571429 0.7 0.71428571 0.72857143 0.74285714 0.75714286 0.77142857 0.78571429 0.8 0.81428571 0.82857143 0.84285714 0.85714286 0.87142857 0.88571429 0.9 0.91428571 0.92857143 0.94285714 0.95714286 0.97142857 0.98571429 1 1 1 1 1 1
  arc A21 (-14.873911, 13.37037) -> (-15.750071, 12.326202) centre (0, 0) ccw
  spline S11 degree 5 poles (-13.998575, 9.494162) (-14.006089, 9.499267) (-14.020968, 9.509672) (-14.042834, 9.52587) (-14.071131, 9.54859) (-14.10533, 9.578527) (-14.138686, 9.609581) (-14.171524, 9.641334) (-14.204082, 9.673474) (-14.236451, 9.70588) (-14.26862, 9.738556) (-14.300516, 9.771583) (-14.33205, 9.805066) (-14.363159, 9.839079) (-14.39384, 9.873623) (-14.424122, 9.908656) (-14.454056, 9.944111) (-14.483697, 9.97992) (-14.513083, 10.016032) (-14.542226, 10.052428) (-14.571122, 10.089111) (-14.599759, 10.126094) (-14.628121, 10.163392) (-14.656202, 10.201013) (-14.684003, 10.238952) (-14.711532, 10.277197) (-14.7388, 10.315731) (-14.76582, 10.35454) (-14.792599, 10.39361) (-14.819141, 10.432935) (-14.845446, 10.472514) (-14.871513, 10.512344) (-14.897342, 10.552427) (-14.922931, 10.59276) (-14.948283, 10.63334) (-14.9734, 10.674162) (-14.998286, 10.71522) (-15.022944, 10.756508) (-15.047376, 10.798023) (-15.071584, 10.83976) (-15.095569, 10.881717) (-15.119331, 10.923891) (-15.142871, 10.966281) (-15.16619, 11.008883) (-15.189289, 11.051696) (-15.212169, 11.094715) (-15.234832, 11.137939) (-15.257278, 11.181365) (-15.279509, 11.224989) (-15.301525, 11.268809) (-15.323328, 11.312823) (-15.344917, 11.357029) (-15.366295, 11.401425) (-15.38746, 11.446008) (-15.408415, 11.490777) (-15.429159, 11.53573) (-15.449693, 11.580863) (-15.470018, 11.626176) (-15.490134, 11.671666) (-15.510043, 11.717332) (-15.529744, 11.763171) (-15.549238, 11.809183) (-15.568525, 11.855365) (-15.587606, 11.901715) (-15.606482, 11.948232) (-15.625151, 11.994914) (-15.643616, 12.041758) (-15.661877, 12.088763) (-15.679933, 12.135927) (-15.697785, 12.18325) (-15.715433, 12.230731) (-15.72939, 12.268841) (-15.739766, 12.297494) (-15.746643, 12.316628) (-15.750071, 12.326202) knots 0 0 0 0 0 0 0.01428571 0.02857143 0.04285714 0.05714286 0.07142857 0.08571429 0.1 0.11428571 0.12857143 0.14285714 0.15714286 0.17142857 0.18571429 0.2 0.21428571 0.22857143 0.24285714 0.25714286 0.27142857 0.28571429 0.3 0.31428571 0.32857143 0.34285714 0.35714286 0.37142857 0.38571429 0.4 0.41428571 0.42857143 0.44285714 0.45714286 0.47142857 0.48571429 0.5 0.51428571 0.52857143 0.54285714 0.55714286 0.57142857 0.58571429 0.6 0.61428571 0.62857143 0.64285714 0.65714286 0.67142857 0.68571429 0.7 0.71428571 0.72857143 0.74285714 0.75714286 0.77142857 0.78571429 0.8 0.81428571 0.82857143 0.84285714 0.85714286 0.87142857 0.88571429 0.9 0.91428571 0.92857143 0.94285714 0.95714286 0.97142857 0.98571429 1 1 1 1 1 1
  line L11 (-13.998575, 9.494162) -> (-13.748372, 9.324199)
  arc A22 (-13.417296, 7.858359) -> (-13.748372, 9.324199) centre (-14.366478, 8.414284) ccw
  arc A23 (-13.417296, 7.858359) -> (-13.514186, 7.690539) centre (0, 0) ccw
  arc A24 (-14.949179, 7.24434) -> (-13.514186, 7.690539) centre (-14.470223, 8.234593) ccw
  line L12 (-14.949179, 7.24434) -> (-15.221473, 7.37604)
  spline S12 degree 5 poles (-15.221473, 7.37604) (-15.229651, 7.379996) (-15.246102, 7.387678) (-15.271063, 7.398516) (-15.304887, 7.411662) (-15.347913, 7.42631) (-15.391484, 7.439671) (-15.435402, 7.452232) (-15.479516, 7.464359) (-15.523765, 7.476189) (-15.568147, 7.487709) (-15.612697, 7.498818) (-15.657461, 7.509386) (-15.702472, 7.519321) (-15.747728, 7.528619) (-15.793208, 7.537328) (-15.838881, 7.545524) (-15.884713, 7.55329) (-15.93068, 7.560683) (-15.976771, 7.567723) (-16.022987, 7.574406) (-16.069334, 7.580715) (-16.115816, 7.586629) (-16.162437, 7.592137) (-16.209194, 7.597244) (-16.256079, 7.601962) (-16.303086, 7.60631) (-16.350205, 7.610305) (-16.39743, 7.613962) (-16.444757, 7.617285) (-16.492186, 7.620276) (-16.539714, 7.622936) (-16.587341, 7.625263) (-16.635065, 7.627257) (-16.682884, 7.628923) (-16.730796, 7.630264) (-16.778796, 7.631287) (-16.826882, 7.631997) (-16.87505, 7.632399) (-16.923299, 7.632495) (-16.971627, 7.632288) (-17.020033, 7.631779) (-17.068513, 7.630971) (-17.117067, 7.629865) (-17.165694, 7.628463) (-17.21439, 7.626767) (-17.263154, 7.624782) (-17.311985, 7.622508) (-17.36088, 7.619948) (-17.409837, 7.617105) (-17.458856, 7.61398) (-17.507934, 7.610574) (-17.557071, 7.606889) (-17.606264, 7.602927) (-17.655512, 7.59869) (-17.704814, 7.594179) (-17.754168, 7.589395) (-17.803573, 7.58434) (-17.853027, 7.579017) (-17.902528, 7.573425) (-17.952077, 7.567567) (-18.001671, 7.561443) (-18.051309, 7.555056) (-18.100991, 7.548405) (-18.150713, 7.541493) (-18.200476, 7.534321) (-18.250276, 7.52689) (-18.300114, 7.519202) (-18.349988, 7.511256) (-18.399897, 7.503055) (-18.44984, 7.494599) (-18.489823, 7.487631) (-18.519825, 7.48229) (-18.539834, 7.478679) (-18.54984, 7.476861) knots 0 0 0 0 0 0 0.01428571 0.02857143 0.04285714 0.05714286 0.07142857 0.08571429 0.1 0.11428571 0.12857143 0.14285714 0.15714286 0.17142857 0.18571429 0.2 0.21428571 0.22857143 0.24285714 0.25714286 0.27142857 0.28571429 0.3 0.31428571 0.32857143 0.34285714 0.35714286 0.37142857 0.38571429 0.4 0.41428571 0.42857143 0.44285714 0.45714286 0.47142857 0.48571429 0.5 0.51428571 0.52857143 0.54285714 0.55714286 0.57142857 0.58571429 0.6 0.61428571 0.62857143 0.64285714 0.65714286 0.67142857 0.68571429 0.7 0.71428571 0.72857143 0.74285714 0.75714286 0.77142857 0.78571429 0.8 0.81428571 0.82857143 0.84285714 0.85714286 0.87142857 0.88571429 0.9 0.91428571 0.92857143 0.94285714 0.95714286 0.97142857 0.98571429 1 1 1 1 1 1
  arc A25 (-18.54984, 7.476861) -> (-19.016035, 6.196) centre (0, 0) ccw
  spline S13 degree 5 poles (-16.401552, 4.133799) (-16.410359, 4.136026) (-16.427899, 4.140716) (-16.453987, 4.148458) (-16.488348, 4.160129) (-16.530723, 4.176564) (-16.572689, 4.194337) (-16.614407, 4.212944) (-16.655995, 4.23201) (-16.697495, 4.251391) (-16.738899, 4.271094) (-16.780167, 4.29122) (-16.821252, 4.311899) (-16.862118, 4.33322) (-16.902763, 4.355187) (-16.943201, 4.37775) (-16.983457, 4.40083) (-17.023557, 4.424341) (-17.063522, 4.448224) (-17.103355, 4.472458) (-17.143055, 4.497046) (-17.182613, 4.522004) (-17.222022, 4.547352) (-17.261277, 4.5731) (-17.300377, 4.599242) (-17.339326, 4.625766) (-17.37813, 4.65265) (-17.416793, 4.679877) (-17.45532, 4.707432) (-17.493711, 4.735308) (-17.531967, 4.763502) (-17.570085, 4.792015) (-17.608065, 4.820847) (-17.645905, 4.849996) (-17.683608, 4.879458) (-17.721172, 4.909227) (-17.7586, 4.939297) (-17.795892, 4.969662) (-17.83305, 5.000317) (-17.870073, 5.031257) (-17.906961, 5.06248) (-17.943714, 5.093984) (-17.980333, 5.125766) (-18.016817, 5.157824) (-18.053165, 5.190154) (-18.089379, 5.222754) (-18.125459, 5.25562) (-18.161403, 5.288749) (-18.197214, 5.322139) (-18.23289, 5.355787) (-18.268431, 5.389689) (-18.303838, 5.423845) (-18.339111, 5.458252) (-18.374248, 5.492908) (-18.409251, 5.52781) (-18.444118, 5.562957) (-18.478851, 5.598346) (-18.513448, 5.633974) (-18.54791, 5.669841) (-18.582236, 5.705943) (-18.616427, 5.74228) (-18.650482, 5.778849) (-18.684402, 5.81565) (-18.718185, 5.852679) (-18.751832, 5.889934) (-18.785342, 5.927415) (-18.818715, 5.965119) (-18.85195, 6.003044) (-18.885049, 6.041189) (-18.918009, 6.079552) (-18.950833, 6.118133) (-18.976982, 6.149171) (-18.996533, 6.172548) (-19.009539, 6.188175) (-19.016035, 6.196) knots 0 0 0 0 0 0 0.01428571 0.02857143 0.04285714 0.05714286 0.07142857 0.08571429 0.1 0.11428571 0.12857143 0.14285714 0.15714286 0.17142857 0.18571429 0.2 0.21428571 0.22857143 0.24285714 0.25714286 0.27142857 0.28571429 0.3 0.31428571 0.32857143 0.34285714 0.35714286 0.37142857 0.38571429 0.4 0.41428571 0.42857143 0.44285714 0.45714286 0.47142857 0.48571429 0.5 0.51428571 0.52857143 0.54285714 0.55714286 0.57142857 0.58571429 0.6 0.61428571 0.62857143 0.64285714 0.65714286 0.67142857 0.68571429 0.7 0.71428571 0.72857143 0.74285714 0.75714286 0.77142857 0.78571429 0.8 0.81428571 0.82857143 0.84285714 0.85714286 0.87142857 0.88571429 0.9 0.91428571 0.92857143 0.94285714 0.95714286 0.97142857 0.98571429 1 1 1 1 1 1
  line L13 (-16.401552, 4.133799) -> (-16.108307, 4.059661)
  arc A26 (-15.295851, 2.795456) -> (-16.108307, 4.059661) centre (-16.377928, 2.993216) ccw
  arc A27 (-15.295851, 2.795456) -> (-15.3295, 2.604619) centre (0, 0) ccw
  arc A28 (-16.525343, 1.694532) -> (-15.3295, 2.604619) centre (-16.413958, 2.788878) ccw
  line L14 (-16.525343, 1.694532) -> (-16.82626, 1.72516)
  spline S14 degree 5 poles (-16.82626, 1.72516) (-16.835298, 1.72608) (-16.853384, 1.727673) (-16.880546, 1.72932) (-16.916827, 1.730104) (-16.962268, 1.729154) (-17.007781, 1.726806) (-17.053347, 1.723589) (-17.098948, 1.719897) (-17.144574, 1.715879) (-17.19022, 1.711525) (-17.235883, 1.706727) (-17.281562, 1.701347) (-17.327256, 1.695289) (-17.372963, 1.688548) (-17.418679, 1.681176) (-17.464401, 1.673257) (-17.510125, 1.664879) (-17.555848, 1.656105) (-17.601568, 1.646956) (-17.647283, 1.637429) (-17.692991, 1.627506) (-17.738693, 1.617166) (-17.784387, 1.606396) (-17.83007, 1.595203) (-17.875742, 1.583601) (-17.9214, 1.57161) (-17.967044, 1.559248) (-18.012672, 1.546532) (-18.058282, 1.533468) (-18.103873, 1.520058) (-18.149445, 1.506301) (-18.194995, 1.492198) (-18.240523, 1.47775) (-18.286029, 1.46296) (-18.331509, 1.447834) (-18.376965, 1.432378) (-18.422393, 1.416599) (-18.467794, 1.400502) (-18.513167, 1.38409) (-18.558509, 1.367366) (-18.603821, 1.350333) (-18.649102, 1.332992) (-18.694349, 1.315346) (-18.739564, 1.297397) (-18.784743, 1.279149) (-18.829888, 1.260605) (-18.874996, 1.241767) (-18.920066, 1.222639) (-18.965099, 1.203222) (-19.010093, 1.18352) (-19.055046, 1.163534) (-19.099959, 1.143266) (-19.144831, 1.122718) (-19.18966, 1.101892) (-19.234445, 1.08079) (-19.279187, 1.059415) (-19.323883, 1.037768) (-19.368534, 1.015851) (-19.413138, 0.993666) (-19.457695, 0.971215) (-19.502203, 0.948498) (-19.546664, 0.925519) (-19.591074, 0.902277) (-19.635434, 0.878776) (-19.679742, 0.855017) (-19.723998, 0.831001) (-19.768201, 0.806731) (-19.812349, 0.782207) (-19.856443, 0.75743) (-19.900483, 0.732402) (-19.935671, 0.712179) (-19.962037, 0.696899) (-19.979604, 0.686663) (-19.988384, 0.681532) knots 0 0 0 0 0 0 0.01428571 0.02857143 0.04285714 0.05714286 0.07142857 0.08571429 0.1 0.11428571 0.12857143 0.14285714 0.15714286 0.17142857 0.18571429 0.2 0.21428571 0.22857143 0.24285714 0.25714286 0.27142857 0.28571429 0.3 0.31428571 0.32857143 0.34285714 0.35714286 0.37142857 0.38571429 0.4 0.41428571 0.42857143 0.44285714 0.45714286 0.47142857 0.48571429 0.5 0.51428571 0.52857143 0.54285714 0.55714286 0.57142857 0.58571429 0.6 0.61428571 0.62857143 0.64285714 0.65714286 0.67142857 0.68571429 0.7 0.71428571 0.72857143 0.74285714 0.75714286 0.77142857 0.78571429 0.8 0.81428571 0.82857143 0.84285714 0.85714286 0.87142857 0.88571429 0.9 0.91428571 0.92857143 0.94285714 0.95714286 0.97142857 0.98571429 1 1 1 1 1 1
  arc A29 (-19.988384, 0.681532) -> (-19.988384, -0.681532) centre (0, 0) ccw
  spline S15 degree 5 poles (-16.82626, -1.72516) (-16.835298, -1.72608) (-16.853384, -1.727673) (-16.880546, -1.72932) (-16.916827, -1.730104) (-16.962268, -1.729154) (-17.007781, -1.726806) (-17.053347, -1.723589) (-17.098948, -1.719897) (-17.144574, -1.715879) (-17.19022, -1.711525) (-17.235883, -1.706727) (-17.281562, -1.701347) (-17.327256, -1.695289) (-17.372963, -1.688548) (-17.418679, -1.681176) (-17.464401, -1.673257) (-17.510125, -1.664879) (-17.555848, -1.656105) (-17.601568, -1.646956) (-17.647283, -1.637429) (-17.692991, -1.627506) (-17.738693, -1.617166) (-17.784387, -1.606396) (-17.83007, -1.595203) (-17.875742, -1.583601) (-17.9214, -1.57161) (-17.967044, -1.559248) (-18.012672, -1.546532) (-18.058282, -1.533468) (-18.103873, -1.520058) (-18.149445, -1.506301) (-18.194995, -1.492198) (-18.240523, -1.47775) (-18.286029, -1.46296) (-18.331509, -1.447834) (-18.376965, -1.432378) (-18.422393, -1.416599) (-18.467794, -1.400502) (-18.513167, -1.38409) (-18.558509, -1.367366) (-18.603821, -1.350333) (-18.649102, -1.332992) (-18.694349, -1.315346) (-18.739564, -1.297397) (-18.784743, -1.279149) (-18.829888, -1.260605) (-18.874996, -1.241767) (-18.920066, -1.222639) (-18.965099, -1.203222) (-19.010093, -1.18352) (-19.055046, -1.163534) (-19.099959, -1.143266) (-19.144831, -1.122718) (-19.18966, -1.101892) (-19.234445, -1.08079) (-19.279187, -1.059415) (-19.323883, -1.037768) (-19.368534, -1.015851) (-19.413138, -0.993666) (-19.457695, -0.971215) (-19.502203, -0.948498) (-19.546664, -0.925519) (-19.591074, -0.902277) (-19.635434, -0.878776) (-19.679742, -0.855017) (-19.723998, -0.831001) (-19.768201, -0.806731) (-19.812349, -0.782207) (-19.856443, -0.75743) (-19.900483, -0.732402) (-19.935671, -0.712179) (-19.962037, -0.696899) (-19.979604, -0.686663) (-19.988384, -0.681532) knots 0 0 0 0 0 0 0.01428571 0.02857143 0.04285714 0.05714286 0.07142857 0.08571429 0.1 0.11428571 0.12857143 0.14285714 0.15714286 0.17142857 0.18571429 0.2 0.21428571 0.22857143 0.24285714 0.25714286 0.27142857 0.28571429 0.3 0.31428571 0.32857143 0.34285714 0.35714286 0.37142857 0.38571429 0.4 0.41428571 0.42857143 0.44285714 0.45714286 0.47142857 0.48571429 0.5 0.51428571 0.52857143 0.54285714 0.55714286 0.57142857 0.58571429 0.6 0.61428571 0.62857143 0.64285714 0.65714286 0.67142857 0.68571429 0.7 0.71428571 0.72857143 0.74285714 0.75714286 0.77142857 0.78571429 0.8 0.81428571 0.82857143 0.84285714 0.85714286 0.87142857 0.88571429 0.9 0.91428571 0.92857143 0.94285714 0.95714286 0.97142857 0.98571429 1 1 1 1 1 1
  line L15 (-16.82626, -1.72516) -> (-16.525343, -1.694532)
  arc A30 (-15.3295, -2.604619) -> (-16.525343, -1.694532) centre (-16.413958, -2.788878) ccw
  arc A31 (-15.3295, -2.604619) -> (-15.295851, -2.795456) centre (0, 0) ccw
  arc A32 (-16.108307, -4.059661) -> (-15.295851, -2.795456) centre (-16.377928, -2.993216) ccw
  line L16 (-16.108307, -4.059661) -> (-16.401552, -4.133799)
  spline S16 degree 5 poles (-16.401552, -4.133799) (-16.410359, -4.136026) (-16.427899, -4.140716) (-16.453987, -4.148458) (-16.488348, -4.160129) (-16.530723, -4.176564) (-16.572689, -4.194337) (-16.614407, -4.212944) (-16.655995, -4.23201) (-16.697495, -4.251391) (-16.738899, -4.271094) (-16.780167, -4.29122) (-16.821252, -4.311899) (-16.862118, -4.33322) (-16.902763, -4.355187) (-16.943201, -4.37775) (-16.983457, -4.40083) (-17.023557, -4.424341) (-17.063522, -4.448224) (-17.103355, -4.472458) (-17.143055, -4.497046) (-17.182613, -4.522004) (-17.222022, -4.547352) (-17.261277, -4.5731) (-17.300377, -4.599242) (-17.339326, -4.625766) (-17.37813, -4.65265) (-17.416793, -4.679877) (-17.45532, -4.707432) (-17.493711, -4.735308) (-17.531967, -4.763502) (-17.570085, -4.792015) (-17.608065, -4.820847) (-17.645905, -4.849996) (-17.683608, -4.879458) (-17.721172, -4.909227) (-17.7586, -4.939297) (-17.795892, -4.969662) (-17.83305, -5.000317) (-17.870073, -5.031257) (-17.906961, -5.06248) (-17.943714, -5.093984) (-17.980333, -5.125766) (-18.016817, -5.157824) (-18.053165, -5.190154) (-18.089379, -5.222754) (-18.125459, -5.25562) (-18.161403, -5.288749) (-18.197214, -5.322139) (-18.23289, -5.355787) (-18.268431, -5.389689) (-18.303838, -5.423845) (-18.339111, -5.458252) (-18.374248, -5.492908) (-18.409251, -5.52781) (-18.444118, -5.562957) (-18.478851, -5.598346) (-18.513448, -5.633974) (-18.54791, -5.669841) (-18.582236, -5.705943) (-18.616427, -5.74228) (-18.650482, -5.778849) (-18.684402, -5.81565) (-18.718185, -5.852679) (-18.751832, -5.889934) (-18.785342, -5.927415) (-18.818715, -5.965119) (-18.85195, -6.003044) (-18.885049, -6.041189) (-18.918009, -6.079552) (-18.950833, -6.118133) (-18.976982, -6.149171) (-18.996533, -6.172548) (-19.009539, -6.188175) (-19.016035, -6.196) knots 0 0 0 0 0 0 0.01428571 0.02857143 0.04285714 0.05714286 0.07142857 0.08571429 0.1 0.11428571 0.12857143 0.14285714 0.15714286 0.17142857 0.18571429 0.2 0.21428571 0.22857143 0.24285714 0.25714286 0.27142857 0.28571429 0.3 0.31428571 0.32857143 0.34285714 0.35714286 0.37142857 0.38571429 0.4 0.41428571 0.42857143 0.44285714 0.45714286 0.47142857 0.48571429 0.5 0.51428571 0.52857143 0.54285714 0.55714286 0.57142857 0.58571429 0.6 0.61428571 0.62857143 0.64285714 0.65714286 0.67142857 0.68571429 0.7 0.71428571 0.72857143 0.74285714 0.75714286 0.77142857 0.78571429 0.8 0.81428571 0.82857143 0.84285714 0.85714286 0.87142857 0.88571429 0.9 0.91428571 0.92857143 0.94285714 0.95714286 0.97142857 0.98571429 1 1 1 1 1 1
  arc A33 (-19.016035, -6.196) -> (-18.54984, -7.476861) centre (0, 0) ccw
  spline S17 degree 5 poles (-15.221473, -7.37604) (-15.229651, -7.379996) (-15.246102, -7.387678) (-15.271063, -7.398516) (-15.304887, -7.411662) (-15.347913, -7.42631) (-15.391484, -7.439671) (-15.435402, -7.452232) (-15.479516, -7.464359) (-15.523765, -7.476189) (-15.568147, -7.487709) (-15.612697, -7.498818) (-15.657461, -7.509386) (-15.702472, -7.519321) (-15.747728, -7.528619) (-15.793208, -7.537328) (-15.838881, -7.545524) (-15.884713, -7.55329) (-15.93068, -7.560683) (-15.976771, -7.567723) (-16.022987, -7.574406) (-16.069334, -7.580715) (-16.115816, -7.586629) (-16.162437, -7.592137) (-16.209194, -7.597244) (-16.256079, -7.601962) (-16.303086, -7.60631) (-16.350205, -7.610305) (-16.39743, -7.613962) (-16.444757, -7.617285) (-16.492186, -7.620276) (-16.539714, -7.622936) (-16.587341, -7.625263) (-16.635065, -7.627257) (-16.682884, -7.628923) (-16.730796, -7.630264) (-16.778796, -7.631287) (-16.826882, -7.631997) (-16.87505, -7.632399) (-16.923299, -7.632495) (-16.971627, -7.632288) (-17.020033, -7.631779) (-17.068513, -7.630971) (-17.117067, -7.629865) (-17.165694, -7.628463) (-17.21439, -7.626767) (-17.263154, -7.624782) (-17.311985, -7.622508) (-17.36088, -7.619948) (-17.409837, -7.617105) (-17.458856, -7.61398) (-17.507934, -7.610574) (-17.557071, -7.606889) (-17.606264, -7.602927) (-17.655512, -7.59869) (-17.704814, -7.594179) (-17.754168, -7.589395) (-17.803573, -7.58434) (-17.853027, -7.579017) (-17.902528, -7.573425) (-17.952077, -7.567567) (-18.001671, -7.561443) (-18.051309, -7.555056) (-18.100991, -7.548405) (-18.150713, -7.541493) (-18.200476, -7.534321) (-18.250276, -7.52689) (-18.300114, -7.519202) (-18.349988, -7.511256) (-18.399897, -7.503055) (-18.44984, -7.494599) (-18.489823, -7.487631) (-18.519825, -7.48229) (-18.539834, -7.478679) (-18.54984, -7.476861) knots 0 0 0 0 0 0 0.01428571 0.02857143 0.04285714 0.05714286 0.07142857 0.08571429 0.1 0.11428571 0.12857143 0.14285714 0.15714286 0.17142857 0.18571429 0.2 0.21428571 0.22857143 0.24285714 0.25714286 0.27142857 0.28571429 0.3 0.31428571 0.32857143 0.34285714 0.35714286 0.37142857 0.38571429 0.4 0.41428571 0.42857143 0.44285714 0.45714286 0.47142857 0.48571429 0.5 0.51428571 0.52857143 0.54285714 0.55714286 0.57142857 0.58571429 0.6 0.61428571 0.62857143 0.64285714 0.65714286 0.67142857 0.68571429 0.7 0.71428571 0.72857143 0.74285714 0.75714286 0.77142857 0.78571429 0.8 0.81428571 0.82857143 0.84285714 0.85714286 0.87142857 0.88571429 0.9 0.91428571 0.92857143 0.94285714 0.95714286 0.97142857 0.98571429 1 1 1 1 1 1
  line L17 (-15.221473, -7.37604) -> (-14.949179, -7.24434)
  arc A34 (-13.514186, -7.690539) -> (-14.949179, -7.24434) centre (-14.470223, -8.234593) ccw
  arc A35 (-13.514186, -7.690539) -> (-13.417296, -7.858359) centre (0, 0) ccw
  arc A36 (-13.748372, -9.324199) -> (-13.417296, -7.858359) centre (-14.366478, -8.414284) ccw
  line L18 (-13.748372, -9.324199) -> (-13.998575, -9.494162)